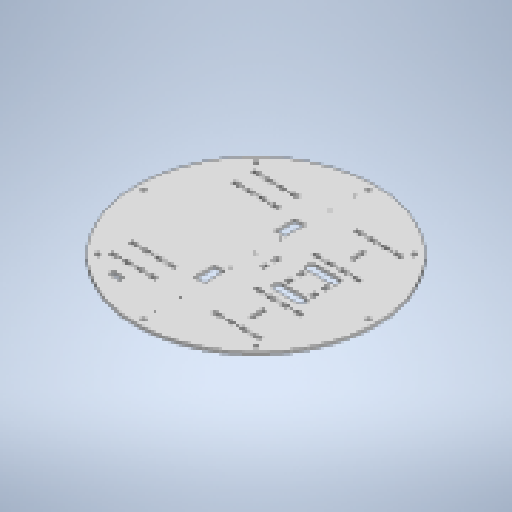
# Autodesk Inventor part: Osn. platform
Saved by Autodesk Inventor 2023.1 (Build 271208000, 208)
## iProperties
Created: 2023-03-13
Part Number: Osn. platform
Material: Типовые
Document SubType Name: Modeling
Designer: User
Density: 1 g/cm^3
Appearance: По умолчанию
Mass: 865.132 g
Surface Area: 3668.91 cm^2
Volume: 865.132 cm^3
Author: User
Autodesk Inventor part; units mm, degrees
(part 1 of 2)
ref_plane "YZ Plane" through (0, 0, 0) normal (1, 0, 0) x (0, 1, 0)
ref_plane "XZ Plane" through (0, 0, 0) normal (0, 1, 0) x (-1, 0, 0)
ref_plane "XY Plane" through (0, 0, 0) normal (0, 0, 1) x (1, 0, 0)
sketch "Основ. платформа" plane through (0, 0, 0) normal (0, 1, 0) x (-1, 0, 0)
  circle A0 centre (0, 0) radius 240
  dimension "d117" = 480
  constraints: 1 centre point, 1 coincident
  measures "d117" diameter of A0
extrude "Осн. платформа" add sketch "Основ. платформа" along normal blind 5
sketch "Эскиз14" plane through (0, 5, 0) normal (0, 1, 0) x (1, 0, 0)
  line L0 (-295.6598, 0) -> (443.256, 0) construction
  line L1 (137.6204, 61.9298) -> (150.9061, 61.9298)
  line L2 (150.9061, 61.9298) -> (150.9061, 55.9298)
  line L3 (137.6204, 55.9298) -> (150.9061, 55.9298)
  line L4 (137.6204, 61.9298) -> (137.6204, 55.9298)
  line L5 (111.049, 61.9298) -> (124.3347, 61.9298)
  line L6 (124.3347, 61.9298) -> (124.3347, 55.9298)
  line L7 (111.049, 55.9298) -> (124.3347, 55.9298)
  line L8 (111.049, 61.9298) -> (111.049, 55.9298)
  line L9 (84.4776, 61.9298) -> (97.7633, 61.9298)
  line L10 (97.7633, 61.9298) -> (97.7633, 55.9298)
  line L11 (84.4776, 55.9298) -> (97.7633, 55.9298)
  line L12 (84.4776, 61.9298) -> (84.4776, 55.9298)
  line L13 (57.9061, 144.9298) -> (71.1919, 144.9298)
  line L14 (71.1919, 144.9298) -> (71.1919, 138.9298)
  line L15 (57.9061, 138.9298) -> (71.1919, 138.9298)
  line L16 (57.9061, 144.9298) -> (57.9061, 138.9298)
  line L17 (84.4776, 144.9298) -> (97.7633, 144.9298)
  line L18 (97.7633, 144.9298) -> (97.7633, 138.9298)
  line L19 (84.4776, 138.9298) -> (97.7633, 138.9298)
  line L20 (84.4776, 144.9298) -> (84.4776, 138.9298)
  line L21 (111.049, 144.9298) -> (124.3347, 144.9298)
  line L22 (124.3347, 144.9298) -> (124.3347, 138.9298)
  line L23 (111.049, 138.9298) -> (124.3347, 138.9298)
  line L24 (111.049, 144.9298) -> (111.049, 138.9298)
  line L25 (137.6204, 144.9298) -> (150.9061, 144.9298)
  line L26 (150.9061, 144.9298) -> (150.9061, 138.9298)
  line L27 (137.6204, 138.9298) -> (150.9061, 138.9298)
  line L28 (137.6204, 144.9298) -> (137.6204, 138.9298)
  line L29 (101.4061, 87.5965) -> (101.4061, 113.2631)
  line L30 (101.4061, 113.2631) -> (107.4061, 113.2631)
  line L31 (107.4061, 113.2631) -> (107.4061, 87.5965)
  line L32 (107.4061, 87.5965) -> (101.4061, 87.5965)
  line L33 (57.9061, 61.9298) -> (71.1919, 61.9298)
  line L34 (71.1919, 61.9298) -> (71.1919, 55.9298)
  line L35 (57.9061, 55.9298) -> (71.1919, 55.9298)
  line L36 (57.9061, 61.9298) -> (57.9061, 55.9298)
  line L37 (-58.1024, 138.9298) -> (-70.9595, 138.9298)
  line L38 (-70.9595, 138.9298) -> (-70.9595, 144.9298)
  line L39 (-58.1024, 144.9298) -> (-70.9595, 144.9298)
  line L40 (-58.1024, 138.9298) -> (-58.1024, 144.9298)
  line L41 (-83.8167, 138.9298) -> (-96.6738, 138.9298)
  line L42 (-96.6738, 138.9298) -> (-96.6738, 144.9298)
  line L43 (-83.8167, 144.9298) -> (-96.6738, 144.9298)
  line L44 (-83.8167, 138.9298) -> (-83.8167, 144.9298)
  line L45 (-109.531, 138.9298) -> (-122.3881, 138.9298)
  line L46 (-122.3881, 138.9298) -> (-122.3881, 144.9298)
  line L47 (-109.531, 144.9298) -> (-122.3881, 144.9298)
  line L48 (-109.531, 138.9298) -> (-109.531, 144.9298)
  line L49 (-135.2452, 140.1831) -> (-148.1024, 140.1831)
  line L50 (-148.1024, 140.1831) -> (-148.1024, 146.1831)
  line L51 (-135.2452, 146.1831) -> (-148.1024, 146.1831)
  line L52 (-135.2452, 140.1831) -> (-135.2452, 146.1831)
  line L53 (-58.1024, 144.9298) -> (-148.1024, 144.9298) construction
  line L54 (-148.1024, 100.7298) -> (-58.1024, 100.7298) construction
  line L55 (137.6204, 138.9298) -> (124.3347, 144.9298) construction
  circle A0 centre (130.9776, 141.9298) radius 1.5
  circle A1 centre (104.2556, 141.9298) radius 1.5
  circle A2 centre (77.5336, 141.9298) radius 1.5
  circle A3 centre (130.9776, 58.9298) radius 1.5
  circle A4 centre (104.2556, 58.9298) radius 1.5
  circle A5 centre (77.5336, 58.9298) radius 1.5
  line L56 (-70.9595, 138.9298) -> (-83.8167, 144.9298) construction
  circle A6 centre (-77.3881, 141.9298) radius 1.5
  circle A7 centre (-103.2571, 141.9298) radius 1.5
  circle A8 centre (-129.1261, 141.9298) radius 1.5
  line L57 (-122.3881, 106.7298) -> (-122.3881, 100.7298)
  line L58 (-109.531, 100.7298) -> (-122.3881, 100.7298)
  line L59 (-109.531, 106.7298) -> (-109.531, 100.7298)
  line L60 (-109.531, 106.7298) -> (-122.3881, 106.7298)
  line L61 (-83.8167, 106.7298) -> (-96.6738, 106.7298)
  line L62 (-70.9595, 106.7298) -> (-70.9595, 100.7298)
  line L63 (-58.1024, 100.7298) -> (-70.9595, 100.7298)
  circle A9 centre (-103.2571, 103.7298) radius 1.5
  circle A10 centre (-129.1261, 103.7298) radius 1.5
  line L64 (-135.2452, 106.7298) -> (-135.2452, 100.7298)
  line L65 (-148.1024, 106.7298) -> (-148.1024, 100.7298)
  line L66 (-135.2452, 100.7298) -> (-148.1024, 100.7298)
  line L67 (-135.2452, 106.7298) -> (-148.1024, 106.7298)
  line L68 (-58.1024, 106.7298) -> (-70.9595, 106.7298)
  line L69 (-58.1024, 106.7298) -> (-58.1024, 100.7298)
  line L70 (-96.6738, 106.7298) -> (-96.6738, 100.7298)
  line L71 (-83.8167, 100.7298) -> (-96.6738, 100.7298)
  line L72 (-83.8167, 106.7298) -> (-83.8167, 100.7298)
  circle A11 centre (-77.3881, 103.7298) radius 1.5
  line L73 (111.049, -61.9298) -> (124.3347, -61.9298)
  line L74 (111.049, -61.9298) -> (111.049, -55.9298)
  line L75 (97.7633, -61.9298) -> (97.7633, -55.9298)
  line L76 (71.1919, -61.9298) -> (71.1919, -55.9298)
  line L77 (57.9061, -61.9298) -> (57.9061, -55.9298)
  line L78 (57.9061, -55.9298) -> (71.1919, -55.9298)
  line L79 (57.9061, -61.9298) -> (71.1919, -61.9298)
  line L80 (107.4061, -87.5965) -> (101.4061, -87.5965)
  line L81 (101.4061, -87.5965) -> (101.4061, -113.2631)
  line L82 (107.4061, -113.2631) -> (107.4061, -87.5965)
  line L83 (57.9061, -138.9298) -> (71.1919, -138.9298)
  line L84 (101.4061, -113.2631) -> (107.4061, -113.2631)
  line L85 (84.4776, -138.9298) -> (97.7633, -138.9298)
  line L86 (84.4776, -144.9298) -> (84.4776, -138.9298)
  line L87 (84.4776, -144.9298) -> (97.7633, -144.9298)
  line L88 (97.7633, -144.9298) -> (97.7633, -138.9298)
  line L89 (111.049, -144.9298) -> (111.049, -138.9298)
  line L90 (111.049, -138.9298) -> (124.3347, -138.9298)
  line L91 (111.049, -144.9298) -> (124.3347, -144.9298)
  line L92 (124.3347, -144.9298) -> (124.3347, -138.9298)
  line L93 (137.6204, -61.9298) -> (150.9061, -61.9298)
  line L94 (150.9061, -61.9298) -> (150.9061, -55.9298)
  line L95 (137.6204, -55.9298) -> (150.9061, -55.9298)
  line L96 (137.6204, -61.9298) -> (137.6204, -55.9298)
  circle A12 centre (130.9776, -58.9298) radius 1.5
  line L97 (137.6204, -144.9298) -> (137.6204, -138.9298)
  line L98 (137.6204, -144.9298) -> (150.9061, -144.9298)
  line L99 (150.9061, -144.9298) -> (150.9061, -138.9298)
  line L100 (137.6204, -138.9298) -> (150.9061, -138.9298)
  line L101 (124.3347, -61.9298) -> (124.3347, -55.9298)
  line L102 (111.049, -55.9298) -> (124.3347, -55.9298)
  line L103 (84.4776, -61.9298) -> (97.7633, -61.9298)
  line L104 (84.4776, -55.9298) -> (97.7633, -55.9298)
  line L105 (84.4776, -61.9298) -> (84.4776, -55.9298)
  line L106 (71.1919, -144.9298) -> (71.1919, -138.9298)
  line L107 (57.9061, -144.9298) -> (71.1919, -144.9298)
  line L108 (57.9061, -144.9298) -> (57.9061, -138.9298)
  line L109 (-58.1024, -100.7298) -> (-70.9595, -100.7298)
  line L110 (-70.9595, -106.7298) -> (-70.9595, -100.7298)
  line L111 (-135.2452, -140.1831) -> (-135.2452, -146.1831)
  line L112 (-135.2452, -140.1831) -> (-148.1024, -140.1831)
  line L113 (-148.1024, -140.1831) -> (-148.1024, -146.1831)
  line L114 (-135.2452, -146.1831) -> (-148.1024, -146.1831)
  line L115 (-96.6738, -138.9298) -> (-96.6738, -144.9298)
  line L116 (-83.8167, -138.9298) -> (-96.6738, -138.9298)
  line L117 (-109.531, -138.9298) -> (-109.531, -144.9298)
  line L118 (-83.8167, -144.9298) -> (-96.6738, -144.9298)
  line L119 (-83.8167, -138.9298) -> (-83.8167, -144.9298)
  circle A13 centre (-129.1261, -141.9298) radius 1.5
  circle A14 centre (-129.1261, -103.7298) radius 1.5
  line L120 (-122.3881, -138.9298) -> (-122.3881, -144.9298)
  line L121 (-122.3881, -106.7298) -> (-122.3881, -100.7298)
  line L122 (-109.531, -144.9298) -> (-122.3881, -144.9298)
  line L123 (-109.531, -100.7298) -> (-122.3881, -100.7298)
  line L124 (-109.531, -138.9298) -> (-122.3881, -138.9298)
  line L125 (-109.531, -106.7298) -> (-122.3881, -106.7298)
  line L126 (-148.1024, -100.7298) -> (-58.1024, -100.7298) construction
  line L127 (-58.1024, -144.9298) -> (-148.1024, -144.9298) construction
  line L128 (-70.9595, -138.9298) -> (-70.9595, -144.9298)
  line L129 (-58.1024, -144.9298) -> (-70.9595, -144.9298)
  line L130 (-109.531, -106.7298) -> (-109.531, -100.7298)
  circle A15 centre (-103.2571, -141.9298) radius 1.5
  line L131 (-135.2452, -106.7298) -> (-135.2452, -100.7298)
  line L132 (-135.2452, -106.7298) -> (-148.1024, -106.7298)
  line L133 (-148.1024, -106.7298) -> (-148.1024, -100.7298)
  line L134 (-135.2452, -100.7298) -> (-148.1024, -100.7298)
  circle A16 centre (77.5336, -58.9298) radius 1.5
  line L135 (-58.1024, -106.7298) -> (-70.9595, -106.7298)
  line L136 (-58.1024, -106.7298) -> (-58.1024, -100.7298)
  line L137 (-58.1024, -138.9298) -> (-70.9595, -138.9298)
  line L138 (-58.1024, -138.9298) -> (-58.1024, -144.9298)
  circle A17 centre (130.9776, -141.9298) radius 1.5
  line L139 (137.6204, -138.9298) -> (124.3347, -144.9298) construction
  circle A18 centre (104.2556, -141.9298) radius 1.5
  circle A19 centre (77.5336, -141.9298) radius 1.5
  circle A20 centre (104.2556, -58.9298) radius 1.5
  line L140 (-70.9595, -138.9298) -> (-83.8167, -144.9298) construction
  circle A21 centre (-77.3881, -141.9298) radius 1.5
  circle A22 centre (-103.2571, -103.7298) radius 1.5
  line L141 (-96.6738, -106.7298) -> (-96.6738, -100.7298)
  line L142 (-83.8167, -100.7298) -> (-96.6738, -100.7298)
  line L143 (-83.8167, -106.7298) -> (-83.8167, -100.7298)
  line L144 (-83.8167, -106.7298) -> (-96.6738, -106.7298)
  circle A23 centre (-77.3881, -103.7298) radius 1.5
  point P0 (0, 0)
  point P1 (-58.1024, 122.8298)
  point P2 (-148.1024, 122.8298)
  point P3 (-148.1024, 100.7298)
  point P4 (-148.1024, -122.8298)
  point P5 (-58.1024, -122.8298)
  point P6 (-148.1024, -100.7298)
  constraints: 290 end point, 85 symmetric about line, 24 centre point, 1 horizontal, 12 other
extrude "Выдавливание9" cut sketch "Эскиз14" against normal up to surface (5 mm away)
sketch "Эскиз16" plane through (0, 5, 0) normal (0, 1, 0) x (1, 0, 0)
  line L0 (-17, -32) -> (-7, -32) construction
  line L1 (-7, -32) -> (-7, -25) construction
  line L2 (-7, -25) -> (-17, -25) construction
  line L3 (-17, -25) -> (-17, -32) construction
  line L4 (66.5859, 0) -> (-61.9521, 0) construction
  line L5 (0, -82.102) -> (0, 52.9941) construction
  line L6 (-17, -75) -> (-17, -82) construction
  line L7 (-17, -82) -> (-7, -82) construction
  line L8 (-7, -82) -> (-7, -75) construction
  line L9 (-7, -75) -> (-17, -75) construction
  line L10 (-17, -125) -> (-17, -132) construction
  line L11 (-17, -132) -> (-7, -132) construction
  line L12 (-7, -132) -> (-7, -125) construction
  line L13 (-7, -125) -> (-17, -125) construction
  line L14 (7, -25) -> (7, -32) construction
  line L15 (7, -32) -> (17, -32) construction
  line L16 (17, -32) -> (17, -25) construction
  line L17 (17, -25) -> (7, -25) construction
  line L18 (7, -75) -> (7, -82) construction
  line L19 (7, -82) -> (17, -82) construction
  line L20 (17, -82) -> (17, -75) construction
  line L21 (17, -75) -> (7, -75) construction
  line L22 (7, -125) -> (7, -132) construction
  line L23 (7, -132) -> (17, -132) construction
  line L24 (17, -132) -> (17, -125) construction
  line L25 (17, -125) -> (7, -125) construction
  line L26 (32, -7) -> (25, -7)
  line L27 (25, -7) -> (25, -17)
  line L28 (25, -17) -> (32, -17)
  line L29 (32, -17) -> (32, -7)
  line L30 (32, -7) -> (25, -17) construction
  line L31 (25, -7) -> (32, -17) construction
  line L32 (75, -17) -> (82, -17)
  line L33 (82, -17) -> (82, -7)
  line L34 (82, -7) -> (75, -7)
  line L35 (75, -7) -> (75, -17)
  line L36 (125, -17) -> (132, -17)
  line L37 (132, -17) -> (132, -7)
  line L38 (132, -7) -> (125, -7)
  line L39 (125, -7) -> (125, -17)
  line L40 (25, 7) -> (32, 7)
  line L41 (32, 7) -> (32, 17)
  line L42 (32, 17) -> (25, 17)
  line L43 (25, 17) -> (25, 7)
  line L44 (75, 7) -> (82, 7)
  line L45 (82, 7) -> (82, 17)
  line L46 (82, 17) -> (75, 17)
  line L47 (75, 17) -> (75, 7)
  line L48 (125, 7) -> (132, 7)
  line L49 (132, 7) -> (132, 17)
  line L50 (132, 17) -> (125, 17)
  line L51 (125, 17) -> (125, 7)
  circle A0 centre (104.2556, -58.9298) radius 1.5 construction
  circle A1 centre (130.9776, -58.9298) radius 1.5 construction
  line L52 (125.6303, -33.4298) -> (77.5364, -33.4298) construction
  line L53 (125.6303, -24.4298) -> (77.5364, -24.4298)
  line L54 (77.5364, -42.4298) -> (125.6303, -42.4298)
  arc A2 (125.6303, -42.4298) -> (125.6303, -24.4298) centre (125.6303, -33.4298) ccw
  arc A3 (77.5364, -24.4298) -> (77.5364, -42.4298) centre (77.5364, -33.4298) ccw
  line L55 (125.6303, 33.4298) -> (77.5364, 33.4298) construction
  line L56 (125.6303, 24.4298) -> (77.5364, 24.4298)
  line L57 (77.5364, 42.4298) -> (125.6303, 42.4298)
  arc A4 (125.6303, 24.4298) -> (125.6303, 42.4298) centre (125.6303, 33.4298) ccw
  arc A5 (77.5364, 42.4298) -> (77.5364, 24.4298) centre (77.5364, 33.4298) ccw
  circle A6 centre (-225.3213, 0) radius 4
  circle A7 centre (-159.3262, -159.3262) radius 4
  circle A8 centre (0, -225.3213) radius 4
  circle A9 centre (159.3262, -159.3262) radius 4
  circle A10 centre (225.3213, 0) radius 4
  circle A11 centre (159.3262, 159.3262) radius 4
  circle A12 centre (0, 225.3213) radius 4
  circle A13 centre (-159.3262, 159.3262) radius 4
  line L58 (-22, 32) -> (22, 32) construction
  line L59 (32, 22) -> (32, -22) construction
  line L60 (22, -32) -> (-22, -32) construction
  line L61 (-32, -22) -> (-32, 22) construction
  line L62 (-32, 32) -> (32, -32) construction
  line L63 (32, 32) -> (-32, -32) construction
  arc A14 (-22, 32) -> (-32, 22) centre (-22, 22) ccw construction
  arc A15 (-32, -22) -> (-22, -32) centre (-22, -22) ccw construction
  arc A16 (22, -32) -> (32, -22) centre (22, -22) ccw construction
  arc A17 (32, 22) -> (22, 32) centre (22, 22) ccw construction
  line L64 (-4.1722, 101.2362) -> (-8.7222, 101.2388) construction
  arc A18 (-22.6837, 81.7061) -> (-22.6574, 81.5943) centre (-22.4337, 81.7059) ccw construction
  line L65 (-22.6574, 81.5943) -> (-22.484, 81.247) construction
  line L66 (-22.484, 81.247) -> (-22.6578, 80.8998) construction
  arc A19 (-22.6578, 80.8998) -> (-22.6843, 80.7881) centre (-22.4343, 80.7879) ccw construction
  line L67 (-22.6843, 80.7881) -> (-22.6876, 75.1971) construction
  arc A20 (-22.6876, 75.1971) -> (-22.4377, 74.9469) centre (-22.4376, 75.1969) ccw construction
  line L68 (-22.4377, 74.9469) -> (-22.0877, 74.9467) construction
  line L69 (-22.0877, 74.9467) -> (-22.0879, 74.5667) construction
  arc A21 (-22.0879, 74.5667) -> (-21.8381, 74.3166) centre (-21.8379, 74.5666) ccw construction
  line L70 (-21.8381, 74.3166) -> (-20.9381, 74.316) construction
  arc A22 (-20.9381, 74.316) -> (-20.6879, 74.5659) centre (-20.9379, 74.566) ccw construction
  line L71 (-20.6879, 74.5659) -> (-20.687, 76.1959) construction
  arc A23 (-20.4368, 76.4457) -> (-20.687, 76.1959) centre (-20.437, 76.1957) ccw construction
  line L72 (-20.4368, 76.4457) -> (-19.291, 76.4451) construction
  arc A24 (-18.5841, 76.1518) -> (-19.291, 76.4451) centre (-19.2916, 75.4451) ccw construction
  line L73 (-18.5841, 76.1518) -> (-17.2736, 74.8397) construction
  arc A25 (-16.6886, 73.4252) -> (-17.2736, 74.8397) centre (-18.6886, 73.4263) ccw construction
  line L74 (-16.6886, 73.4252) -> (-16.6896, 71.7026) construction
  arc A26 (-16.6896, 71.7026) -> (-16.6633, 71.5907) centre (-16.4396, 71.7024) ccw construction
  line L75 (-16.6633, 71.5907) -> (-16.4899, 71.2434) construction
  line L76 (-16.4899, 71.2434) -> (-16.6637, 70.8963) construction
  arc A27 (-16.6637, 70.8963) -> (-16.6902, 70.7845) centre (-16.4402, 70.7843) ccw construction
  line L77 (-16.6902, 70.7845) -> (-16.6912, 69.0619) construction
  arc A28 (-17.2778, 67.648) -> (-16.6912, 69.0619) centre (-18.6912, 69.0631) ccw construction
  line L78 (-17.2778, 67.648) -> (-18.5898, 66.3375) construction
  arc A29 (-19.2971, 66.0451) -> (-18.5898, 66.3375) centre (-19.2965, 67.0451) ccw construction
  line L79 (-19.2971, 66.0451) -> (-20.443, 66.0457) construction
  arc A30 (-20.6928, 66.2959) -> (-20.443, 66.0457) centre (-20.4428, 66.2957) ccw construction
  line L80 (-20.6928, 66.2959) -> (-20.6919, 67.9259) construction
  arc A31 (-20.6919, 67.9259) -> (-20.9417, 68.176) centre (-20.9419, 67.926) ccw construction
  line L81 (-20.9417, 68.176) -> (-21.8417, 68.1766) construction
  arc A32 (-21.8417, 68.1766) -> (-22.0919, 67.9267) centre (-21.8419, 67.9266) ccw construction
  line L82 (-22.0919, 67.9267) -> (-22.0921, 67.5467) construction
  line L83 (-22.0921, 67.5467) -> (-22.4421, 67.5469) construction
  arc A33 (-22.4421, 67.5469) -> (-22.6922, 67.2971) centre (-22.4422, 67.2969) ccw construction
  line L84 (-22.6922, 67.2971) -> (-22.6949, 62.7471) construction
  arc A34 (-22.6949, 62.7471) -> (-21.1958, 61.2462) centre (-21.1949, 62.7462) ccw construction
  line L85 (-21.1958, 61.2462) -> (-16.6458, 61.2435) construction
  arc A35 (-16.6458, 61.2435) -> (-16.3956, 61.4934) centre (-16.6456, 61.4935) ccw construction
  line L86 (-16.3956, 61.4934) -> (-16.3954, 61.8434) construction
  line L87 (-16.3954, 61.8434) -> (-16.0154, 61.8431) construction
  arc A36 (-16.0154, 61.8431) -> (-15.7653, 62.093) centre (-16.0153, 62.0931) ccw construction
  line L88 (-15.7653, 62.093) -> (-15.7648, 62.993) construction
  arc A37 (-15.7648, 62.993) -> (-15.9008, 63.2431) centre (-16.0623, 62.9932) ccw construction
  line L89 (-15.9008, 63.2431) -> (-17.6446, 63.2441) construction
  arc A38 (-17.8945, 63.4942) -> (-17.6446, 63.2441) centre (-17.6445, 63.4941) ccw construction
  line L90 (-17.8945, 63.4942) -> (-17.8938, 64.6401) construction
  arc A39 (-17.6005, 65.347) -> (-17.8938, 64.6401) centre (-16.8938, 64.6395) ccw construction
  line L91 (-17.6005, 65.347) -> (-16.2884, 66.6575) construction
  arc A40 (-14.8739, 67.2425) -> (-16.2884, 66.6575) centre (-14.875, 65.2425) ccw construction
  line L92 (-14.8739, 67.2425) -> (-13.1513, 67.2414) construction
  arc A41 (-13.1513, 67.2414) -> (-13.0394, 67.2678) centre (-13.1511, 67.4914) ccw construction
  line L93 (-13.0394, 67.2678) -> (-12.6921, 67.4412) construction
  line L94 (-12.6921, 67.4412) -> (-12.345, 67.2674) construction
  arc A42 (-12.345, 67.2674) -> (-12.2332, 67.2409) centre (-12.2331, 67.4909) ccw construction
  line L95 (-12.2332, 67.2409) -> (-10.5106, 67.2399) construction
  arc A43 (-9.0968, 66.6533) -> (-10.5106, 67.2399) centre (-10.5118, 65.2399) ccw construction
  line L96 (-9.0968, 66.6533) -> (-7.7863, 65.3412) construction
  arc A44 (-7.4938, 64.6339) -> (-7.7863, 65.3412) centre (-8.4938, 64.6345) ccw construction
  line L97 (-7.4938, 64.6339) -> (-7.4945, 63.4881) construction
  arc A45 (-7.7446, 63.2383) -> (-7.4945, 63.4881) centre (-7.7445, 63.4883) ccw construction
  line L98 (-7.7446, 63.2383) -> (-9.5773, 63.2393) construction
  arc A46 (-9.5773, 63.2393) -> (-9.6248, 62.9894) centre (-8.9399, 62.989) ccw construction
  line L99 (-9.6248, 62.9894) -> (-9.6253, 62.0894) construction
  arc A47 (-9.6253, 62.0894) -> (-9.3754, 61.8392) centre (-9.3753, 62.0892) ccw construction
  line L100 (-9.3754, 61.8392) -> (-8.9954, 61.839) construction
  line L101 (-8.9954, 61.839) -> (-8.9956, 61.489) construction
  arc A48 (-8.9956, 61.489) -> (-8.7458, 61.2389) centre (-8.7456, 61.4889) ccw construction
  line L102 (-8.7458, 61.2389) -> (-4.1958, 61.2362) construction
  arc A49 (-4.1958, 61.2362) -> (-2.6949, 62.7353) centre (-4.1949, 62.7362) ccw construction
  line L103 (-2.6949, 62.7353) -> (-2.6922, 67.2853) construction
  arc A50 (-2.6922, 67.2853) -> (-2.9421, 67.5354) centre (-2.9422, 67.2854) ccw construction
  line L104 (-2.9421, 67.5354) -> (-3.2921, 67.5356) construction
  line L105 (-3.2921, 67.5356) -> (-3.2919, 67.9156) construction
  arc A51 (-3.2919, 67.9156) -> (-3.5417, 68.1658) centre (-3.5419, 67.9158) ccw construction
  line L106 (-3.5417, 68.1658) -> (-4.4417, 68.1663) construction
  arc A52 (-4.4417, 68.1663) -> (-4.6919, 67.9165) centre (-4.4419, 67.9163) ccw construction
  line L107 (-4.6919, 67.9165) -> (-4.6928, 66.2865) construction
  arc A53 (-4.943, 66.0366) -> (-4.6928, 66.2865) centre (-4.9428, 66.2866) ccw construction
  line L108 (-4.943, 66.0366) -> (-6.0888, 66.0373) construction
  arc A54 (-6.7957, 66.3306) -> (-6.0888, 66.0373) centre (-6.0882, 67.0373) ccw construction
  line L109 (-6.7957, 66.3306) -> (-8.1062, 67.6426) construction
  arc A55 (-8.6912, 69.0572) -> (-8.1062, 67.6426) centre (-6.6912, 69.056) ccw construction
  line L110 (-8.6912, 69.0572) -> (-8.6902, 70.7798) construction
  arc A56 (-8.6902, 70.7798) -> (-8.7165, 70.8916) centre (-8.9402, 70.78) ccw construction
  line L111 (-8.7165, 70.8916) -> (-8.8899, 71.2389) construction
  line L112 (-8.8899, 71.2389) -> (-8.7161, 71.586) construction
  arc A57 (-8.7161, 71.586) -> (-8.6896, 71.6978) centre (-8.9396, 71.698) ccw construction
  line L113 (-8.6896, 71.6978) -> (-8.6886, 73.4204) construction
  arc A58 (-8.102, 74.8343) -> (-8.6886, 73.4204) centre (-6.6886, 73.4193) ccw construction
  line L114 (-8.102, 74.8343) -> (-6.7899, 76.1448) construction
  arc A59 (-6.0827, 76.4373) -> (-6.7899, 76.1448) centre (-6.0833, 75.4373) ccw construction
  line L115 (-6.0827, 76.4373) -> (-4.9368, 76.4366) construction
  arc A60 (-4.687, 76.1865) -> (-4.9368, 76.4366) centre (-4.937, 76.1866) ccw construction
  line L116 (-4.687, 76.1865) -> (-4.6879, 74.5565) construction
  arc A61 (-4.6879, 74.5565) -> (-4.4381, 74.3063) centre (-4.4379, 74.5563) ccw construction
  line L117 (-4.4381, 74.3063) -> (-3.5381, 74.3058) construction
  arc A62 (-3.5381, 74.3058) -> (-3.2879, 74.5556) centre (-3.5379, 74.5558) ccw construction
  line L118 (-3.2879, 74.5556) -> (-3.2877, 74.9356) construction
  line L119 (-3.2877, 74.9356) -> (-2.9377, 74.9354) construction
  arc A63 (-2.9377, 74.9354) -> (-2.6876, 75.1853) centre (-2.9376, 75.1854) ccw construction
  line L120 (-2.6876, 75.1853) -> (-2.6843, 80.7763) construction
  arc A64 (-2.6843, 80.7763) -> (-2.7106, 80.8881) centre (-2.9343, 80.7764) ccw construction
  line L121 (-2.7106, 80.8881) -> (-2.884, 81.2354) construction
  line L122 (-2.884, 81.2354) -> (-2.7102, 81.5825) construction
  arc A65 (-2.7102, 81.5825) -> (-2.6837, 81.6943) centre (-2.9337, 81.6944) ccw construction
  line L123 (-2.6837, 81.6943) -> (-2.6804, 87.2853) construction
  arc A66 (-2.6804, 87.2853) -> (-2.9303, 87.5354) centre (-2.9304, 87.2854) ccw construction
  line L124 (-2.9303, 87.5354) -> (-3.2803, 87.5356) construction
  line L125 (-3.2803, 87.5356) -> (-3.2801, 87.9156) construction
  arc A67 (-3.2801, 87.9156) -> (-3.5299, 88.1658) centre (-3.5301, 87.9158) ccw construction
  line L126 (-3.5299, 88.1658) -> (-4.4299, 88.1663) construction
  arc A68 (-4.4299, 88.1663) -> (-4.6801, 87.9165) centre (-4.4301, 87.9163) ccw construction
  line L127 (-4.6801, 87.9165) -> (-4.681, 86.2865) construction
  arc A69 (-4.9312, 86.0366) -> (-4.681, 86.2865) centre (-4.931, 86.2866) ccw construction
  line L128 (-4.9312, 86.0366) -> (-6.077, 86.0373) construction
  arc A70 (-6.7839, 86.3306) -> (-6.077, 86.0373) centre (-6.0764, 87.0373) ccw construction
  line L129 (-6.7839, 86.3306) -> (-8.0944, 87.6426) construction
  arc A71 (-8.6794, 89.0572) -> (-8.0944, 87.6426) centre (-6.6794, 89.056) ccw construction
  line L130 (-8.6794, 89.0572) -> (-8.6784, 90.7798) construction
  arc A72 (-8.6784, 90.7798) -> (-8.7047, 90.8916) centre (-8.9284, 90.7799) ccw construction
  line L131 (-8.7047, 90.8916) -> (-8.8781, 91.2389) construction
  line L132 (-8.8781, 91.2389) -> (-8.7043, 91.586) construction
  arc A73 (-8.7043, 91.586) -> (-8.6778, 91.6978) centre (-8.9278, 91.698) ccw construction
  line L133 (-8.6778, 91.6978) -> (-8.6768, 93.4204) construction
  arc A74 (-8.0902, 94.8343) -> (-8.6768, 93.4204) centre (-6.6768, 93.4193) ccw construction
  line L134 (-8.0902, 94.8343) -> (-6.7782, 96.1448) construction
  arc A75 (-6.0709, 96.4373) -> (-6.7782, 96.1448) centre (-6.0715, 95.4373) ccw construction
  line L135 (-6.0709, 96.4373) -> (-4.925, 96.4366) construction
  arc A76 (-4.6752, 96.1865) -> (-4.925, 96.4366) centre (-4.9252, 96.1866) ccw construction
  line L136 (-4.6752, 96.1865) -> (-4.6761, 94.5565) construction
  arc A77 (-4.6761, 94.5565) -> (-4.4263, 94.3063) centre (-4.4261, 94.5563) ccw construction
  line L137 (-4.4263, 94.3063) -> (-3.5263, 94.3058) construction
  arc A78 (-3.5263, 94.3058) -> (-3.2761, 94.5556) centre (-3.5261, 94.5558) ccw construction
  line L138 (-3.2761, 94.5556) -> (-3.2759, 94.9356) construction
  line L139 (-3.2759, 94.9356) -> (-2.9259, 94.9354) construction
  arc A79 (-2.9259, 94.9354) -> (-2.6758, 95.1853) centre (-2.9258, 95.1854) ccw construction
  line L140 (-2.6758, 95.1853) -> (-2.6731, 99.7353) construction
  arc A80 (-2.6731, 99.7353) -> (-4.1722, 101.2362) centre (-4.1731, 99.7362) ccw construction
  line L141 (-4.1722, 101.2362) -> (-8.7222, 101.2388) construction
  arc A81 (-8.7222, 101.2388) -> (-8.9723, 100.989) centre (-8.7223, 100.9888) ccw construction
  line L142 (-8.9723, 100.989) -> (-8.9726, 100.639) construction
  line L143 (-8.9726, 100.639) -> (-9.3526, 100.6392) construction
  arc A82 (-9.3526, 100.6392) -> (-9.6027, 100.3894) centre (-9.3527, 100.3892) ccw construction
  line L144 (-9.6027, 100.3894) -> (-9.6032, 99.4894) construction
  arc A83 (-9.6032, 99.4894) -> (-9.3534, 99.2392) centre (-9.3532, 99.4892) ccw construction
  line L145 (-9.3534, 99.2392) -> (-7.7234, 99.2383) construction
  arc A84 (-7.4735, 98.9881) -> (-7.7234, 99.2383) centre (-7.7235, 98.9883) ccw construction
  line L146 (-7.4735, 98.9881) -> (-7.4742, 97.8423) construction
  arc A85 (-7.7675, 97.1353) -> (-7.4742, 97.8423) centre (-8.4742, 97.8429) ccw construction
  line L147 (-7.7675, 97.1353) -> (-9.0796, 95.8248) construction
  arc A86 (-10.4941, 95.2399) -> (-9.0796, 95.8248) centre (-10.4929, 97.2399) ccw construction
  line L148 (-10.4941, 95.2399) -> (-12.2167, 95.2409) construction
  arc A87 (-12.2167, 95.2409) -> (-12.3285, 95.2146) centre (-12.2169, 94.9909) ccw construction
  line L149 (-12.3285, 95.2146) -> (-12.6759, 95.0412) construction
  line L150 (-12.6759, 95.0412) -> (-13.023, 95.215) construction
  arc A88 (-13.023, 95.215) -> (-13.1348, 95.2414) centre (-13.1349, 94.9914) ccw construction
  line L151 (-13.1348, 95.2414) -> (-14.8574, 95.2425) construction
  arc A89 (-16.2712, 95.8291) -> (-14.8574, 95.2425) centre (-14.8562, 97.2425) ccw construction
  line L152 (-16.2712, 95.8291) -> (-17.5817, 97.1411) construction
  arc A90 (-17.8742, 97.8484) -> (-17.5817, 97.1411) centre (-16.8742, 97.8478) ccw construction
  line L153 (-17.8742, 97.8484) -> (-17.8735, 98.9942) construction
  arc A91 (-17.6234, 99.2441) -> (-17.8735, 98.9942) centre (-17.6235, 98.9941) ccw construction
  line L154 (-17.6234, 99.2441) -> (-15.9934, 99.2431) construction
  arc A92 (-15.9934, 99.2431) -> (-15.7432, 99.493) centre (-15.9932, 99.4931) ccw construction
  line L155 (-15.7432, 99.493) -> (-15.7427, 100.393) construction
  arc A93 (-15.7427, 100.393) -> (-15.9926, 100.6431) centre (-15.9927, 100.3931) ccw construction
  line L156 (-15.9926, 100.6431) -> (-16.3726, 100.6434) construction
  line L157 (-16.3726, 100.6434) -> (-16.3723, 100.9934) construction
  arc A94 (-16.3723, 100.9934) -> (-16.4557, 101.2434) centre (-16.7884, 100.9936) ccw construction
  line L158 (-16.4557, 101.2434) -> (-21.5905, 101.2464) construction
  arc A95 (-21.5905, 101.2464) -> (-22.6731, 99.7471) centre (-21.0922, 99.7461) ccw construction
  line L159 (-22.6731, 99.7471) -> (-22.6758, 95.1971) construction
  arc A96 (-22.6758, 95.1971) -> (-22.4259, 94.9469) centre (-22.4258, 95.1969) ccw construction
  line L160 (-22.4259, 94.9469) -> (-22.0759, 94.9467) construction
  line L161 (-22.0759, 94.9467) -> (-22.0761, 94.5667) construction
  arc A97 (-22.0761, 94.5667) -> (-21.8263, 94.3166) centre (-21.8261, 94.5666) ccw construction
  line L162 (-21.8263, 94.3166) -> (-20.9263, 94.316) construction
  arc A98 (-20.9263, 94.316) -> (-20.6761, 94.5659) centre (-20.9261, 94.566) ccw construction
  line L163 (-20.6761, 94.5659) -> (-20.6752, 96.1959) construction
  arc A99 (-20.425, 96.4457) -> (-20.6752, 96.1959) centre (-20.4252, 96.1957) ccw construction
  line L164 (-20.425, 96.4457) -> (-19.2792, 96.4451) construction
  arc A100 (-18.5723, 96.1518) -> (-19.2792, 96.4451) centre (-19.2798, 95.4451) ccw construction
  line L165 (-18.5723, 96.1518) -> (-17.2618, 94.8397) construction
  arc A101 (-16.6768, 93.4252) -> (-17.2618, 94.8397) centre (-18.6768, 93.4263) ccw construction
  line L166 (-16.6768, 93.4252) -> (-16.6778, 91.7026) construction
  arc A102 (-16.6778, 91.7026) -> (-16.6515, 91.5907) centre (-16.4278, 91.7024) ccw construction
  line L167 (-16.6515, 91.5907) -> (-16.4781, 91.2434) construction
  line L168 (-16.4781, 91.2434) -> (-16.6519, 90.8963) construction
  arc A103 (-16.6519, 90.8963) -> (-16.6784, 90.7845) centre (-16.4284, 90.7844) ccw construction
  line L169 (-16.6784, 90.7845) -> (-16.6794, 89.0619) construction
  arc A104 (-17.266, 87.648) -> (-16.6794, 89.0619) centre (-18.6794, 89.0631) ccw construction
  line L170 (-17.266, 87.648) -> (-18.5781, 86.3375) construction
  arc A105 (-19.2853, 86.0451) -> (-18.5781, 86.3375) centre (-19.2847, 87.0451) ccw construction
  line L171 (-19.2853, 86.0451) -> (-20.4312, 86.0457) construction
  arc A106 (-20.681, 86.2959) -> (-20.4312, 86.0457) centre (-20.431, 86.2957) ccw construction
  line L172 (-20.681, 86.2959) -> (-20.6801, 87.9259) construction
  arc A107 (-20.6801, 87.9259) -> (-20.9299, 88.176) centre (-20.9301, 87.926) ccw construction
  line L173 (-20.9299, 88.176) -> (-21.8299, 88.1766) construction
  arc A108 (-21.8299, 88.1766) -> (-22.0801, 87.9267) centre (-21.8301, 87.9266) ccw construction
  line L174 (-22.0801, 87.9267) -> (-22.0803, 87.5467) construction
  line L175 (-22.0803, 87.5467) -> (-22.4303, 87.5469) construction
  arc A109 (-22.4303, 87.5469) -> (-22.6804, 87.2971) centre (-22.4304, 87.2969) ccw construction
  line L176 (-22.6804, 87.2971) -> (-22.6837, 81.7061) construction
  line L177 (-20.586, 77.8958) -> (-18.6895, 77.8947) construction
  arc A110 (-21.1856, 78.4962) -> (-20.586, 77.8958) centre (-20.5856, 78.4958) ccw construction
  line L178 (-21.1846, 80.1692) -> (-21.1856, 78.4962) construction
  arc A111 (-21.1846, 80.1692) -> (-21.1834, 82.3232) centre (-23.984, 81.2478) ccw construction
  line L179 (-21.1824, 83.9962) -> (-21.1834, 82.3232) construction
  arc A112 (-20.582, 84.5958) -> (-21.1824, 83.9962) centre (-20.5824, 83.9958) ccw construction
  line L180 (-18.6856, 84.5947) -> (-20.582, 84.5958) construction
  arc A113 (-18.6856, 84.5947) -> (-17.9783, 84.8872) centre (-18.685, 85.5947) ccw construction
  line L181 (-15.9129, 86.9502) -> (-17.9783, 84.8872) construction
  arc A114 (-15.2056, 87.2427) -> (-15.9129, 86.9502) centre (-15.2062, 86.2427) ccw construction
  line L182 (-10.1553, 87.2397) -> (-15.2056, 87.2427) construction
  arc A115 (-9.4484, 86.9464) -> (-10.1553, 87.2397) centre (-10.1559, 86.2397) ccw construction
  line L183 (-7.3854, 84.8809) -> (-9.4484, 86.9464) construction
  arc A116 (-7.3854, 84.8809) -> (-6.6785, 84.5876) centre (-6.6779, 85.5877) ccw construction
  line L184 (-4.782, 84.5865) -> (-6.6785, 84.5876) construction
  arc A117 (-4.1824, 83.9862) -> (-4.782, 84.5865) centre (-4.7824, 83.9865) ccw construction
  line L185 (-4.1834, 82.3132) -> (-4.1824, 83.9862) construction
  arc A118 (-4.1834, 82.3132) -> (-4.1846, 80.1591) centre (-1.384, 81.2345) ccw construction
  line L186 (-4.1856, 78.4862) -> (-4.1846, 80.1591) construction
  arc A119 (-4.786, 77.8865) -> (-4.1856, 78.4862) centre (-4.7856, 78.4865) ccw construction
  line L187 (-6.6824, 77.8876) -> (-4.786, 77.8865) construction
  arc A120 (-6.6824, 77.8876) -> (-7.3897, 77.5952) centre (-6.683, 76.8876) ccw construction
  line L188 (-9.4551, 75.5322) -> (-7.3897, 77.5952) construction
  arc A121 (-10.1624, 75.2397) -> (-9.4551, 75.5322) centre (-10.1618, 76.2397) ccw construction
  line L189 (-15.2127, 75.2427) -> (-10.1624, 75.2397) construction
  arc A122 (-15.9196, 75.536) -> (-15.2127, 75.2427) centre (-15.2121, 76.2427) ccw construction
  line L190 (-17.9826, 77.6014) -> (-15.9196, 75.536) construction
  arc A123 (-17.9826, 77.6014) -> (-18.6895, 77.8947) centre (-18.6901, 76.8947) ccw construction
  arc A124 (-10.3229, 70.4366) -> (-10.3219, 69.7902) centre (-9.3761, 70.1148) ccw construction
  arc A125 (-11.2417, 68.8715) -> (-10.3219, 69.7902) centre (-10.7818, 69.3309) ccw construction
  arc A126 (-11.2417, 68.8715) -> (-11.8881, 68.8732) centre (-11.5674, 67.926) ccw construction
  arc A127 (-13.4944, 68.8742) -> (-11.8881, 68.8732) centre (-12.6899, 71.2412) ccw construction
  arc A128 (-13.4944, 68.8742) -> (-14.1409, 68.8732) centre (-13.8163, 67.9274) ccw construction
  arc A129 (-15.0596, 69.793) -> (-14.1409, 68.8732) centre (-14.6002, 69.3331) ccw construction
  arc A130 (-15.0596, 69.793) -> (-15.0578, 70.4394) centre (-16.005, 70.1187) ccw construction
  arc A131 (-15.0569, 72.0457) -> (-15.0578, 70.4394) centre (-12.6899, 71.2412) ccw construction
  arc A132 (-15.0569, 72.0457) -> (-15.0578, 72.6921) centre (-16.0037, 72.3675) ccw construction
  arc A133 (-14.1381, 73.6108) -> (-15.0578, 72.6921) centre (-14.598, 73.1515) ccw construction
  arc A134 (-14.1381, 73.6108) -> (-13.4916, 73.6091) centre (-13.8123, 74.5563) ccw construction
  arc A135 (-11.8853, 73.6082) -> (-13.4916, 73.6091) centre (-12.6899, 71.2412) ccw construction
  arc A136 (-11.8853, 73.6082) -> (-11.2389, 73.6091) centre (-11.5635, 74.555) ccw construction
  arc A137 (-10.3202, 72.6893) -> (-11.2389, 73.6091) centre (-10.7796, 73.1492) ccw construction
  arc A138 (-10.3202, 72.6893) -> (-10.3219, 72.0429) centre (-9.3748, 72.3636) ccw construction
  arc A139 (-10.3229, 70.4366) -> (-10.3219, 72.0429) centre (-12.6899, 71.2412) ccw construction
  arc A140 (-14.1263, 93.6108) -> (-13.4799, 93.6091) centre (-13.8006, 94.5563) ccw construction
  arc A141 (-11.8736, 93.6082) -> (-13.4799, 93.6091) centre (-12.6781, 91.2412) ccw construction
  arc A142 (-11.8736, 93.6082) -> (-11.2271, 93.6091) centre (-11.5517, 94.555) ccw construction
  arc A143 (-10.3084, 92.6893) -> (-11.2271, 93.6091) centre (-10.7678, 93.1492) ccw construction
  arc A144 (-10.3084, 92.6893) -> (-10.3101, 92.0429) centre (-9.363, 92.3636) ccw construction
  arc A145 (-10.3111, 90.4366) -> (-10.3101, 92.0429) centre (-12.6781, 91.2412) ccw construction
  arc A146 (-10.3111, 90.4366) -> (-10.3101, 89.7902) centre (-9.3643, 90.1148) ccw construction
  arc A147 (-11.2299, 88.8715) -> (-10.3101, 89.7902) centre (-10.77, 89.3309) ccw construction
  arc A148 (-11.2299, 88.8715) -> (-11.8763, 88.8732) centre (-11.5556, 87.926) ccw construction
  arc A149 (-13.4826, 88.8742) -> (-11.8763, 88.8732) centre (-12.6781, 91.2412) ccw construction
  arc A150 (-13.4826, 88.8742) -> (-14.1291, 88.8732) centre (-13.8045, 87.9274) ccw construction
  arc A151 (-15.0478, 89.793) -> (-14.1291, 88.8732) centre (-14.5884, 89.3331) ccw construction
  arc A152 (-15.0478, 89.793) -> (-15.046, 90.4394) centre (-15.9932, 90.1187) ccw construction
  arc A153 (-15.0451, 92.0457) -> (-15.046, 90.4394) centre (-12.6781, 91.2412) ccw construction
  arc A154 (-15.0451, 92.0457) -> (-15.0461, 92.6921) centre (-15.9919, 92.3675) ccw construction
  arc A155 (-14.1263, 93.6108) -> (-15.0461, 92.6921) centre (-14.5862, 93.1515) ccw construction
  line L191 (-57.9836, 100.7939) -> (-57.9765, 106.7939) projected
  line L192 (-70.8407, 100.8091) -> (-57.9836, 100.7939) projected
  line L193 (-58.1024, 100.7298) -> (-70.9595, 100.7298) projected
  line L194 (-70.9595, 100.7298) -> (-2.6725, 100.7298) construction
  line L195 (-70.9595, 100.7298) -> (-2.6725, 100.7298) construction
  line L196 (-22.6725, 60.7298) -> (-2.6725, 60.7298)
  line L197 (-2.6725, 60.7298) -> (-2.6725, 100.7298)
  line L198 (-2.6725, 100.7298) -> (-22.6725, 100.7298)
  line L199 (-22.6725, 100.7298) -> (-22.6725, 60.7298)
  line L200 (-22.6725, -60.7298) -> (-2.6725, -60.7298)
  line L201 (-2.6725, -60.7298) -> (-2.6725, -100.7298)
  line L202 (-2.6725, -100.7298) -> (-22.6725, -100.7298)
  line L203 (-22.6725, -100.7298) -> (-22.6725, -60.7298)
  line L204 (17.3275, -173.8636) -> (17.3275, 176.1364) construction
  line L205 (-22.6725, -173.8636) -> (-22.6725, 176.1364) construction
  line L206 (17.3275, -173.8636) -> (-22.6725, 176.1364) construction
  circle A156 centre (-2.6725, 1.1364) radius 1.55
  circle A157 centre (-2.6725, 51.1364) radius 1.55
  circle A158 centre (-2.6725, 101.1364) radius 1.55
  circle A159 centre (-2.6725, 151.1364) radius 1.55
  circle A160 centre (-2.6725, 201.1364) radius 1.55
  circle A161 centre (-2.6725, -48.8636) radius 1.55
  circle A162 centre (-2.6725, 1.1364) radius 1.55
  circle A163 centre (-2.6725, 51.1364) radius 1.55
  circle A164 centre (-2.6725, 101.1364) radius 1.55
  circle A165 centre (-2.6725, 151.1364) radius 1.55
  circle A166 centre (-2.6725, -98.8636) radius 1.55
  circle A167 centre (-2.6725, -48.8636) radius 1.55
  circle A168 centre (-2.6725, 1.1364) radius 1.55
  circle A169 centre (-2.6725, 51.1364) radius 1.55
  circle A170 centre (-2.6725, 101.1364) radius 1.55
  circle A171 centre (-2.6725, -148.8636) radius 1.55
  circle A172 centre (-2.6725, -98.8636) radius 1.55
  circle A173 centre (-2.6725, -48.8636) radius 1.55
  circle A174 centre (-2.6725, 1.1364) radius 1.55
  circle A175 centre (-2.6725, 51.1364) radius 1.55
  circle A176 centre (-2.6725, -198.8636) radius 1.55
  circle A177 centre (-2.6725, -148.8636) radius 1.55
  circle A178 centre (-2.6725, -98.8636) radius 1.55
  circle A179 centre (-2.6725, -48.8636) radius 1.55
  circle A180 centre (-2.6725, 1.1364) radius 1.55
  line L207 (-113.1024, -174.1661) -> (-113.1024, -179.1661) construction
  line L208 (-93.1024, -179.1661) -> (-113.1024, -179.1661) construction
  line L209 (-93.1024, -174.1661) -> (-113.1024, -174.1661) construction
  circle A181 centre (104.2556, -141.9298) radius 1.5 projected
  line L210 (71.1919, -138.9298) -> (71.1919, -144.9298) projected
  line L211 (71.1919, -144.9298) -> (57.9061, -144.9298) projected
  line L212 (57.9061, -144.9298) -> (57.9061, -138.9298) projected
  line L213 (57.9061, -138.9298) -> (71.1919, -138.9298) projected
  line L214 (97.7633, -55.9298) -> (97.7633, -61.9298) projected
  line L215 (97.7633, -61.9298) -> (84.4776, -61.9298) projected
  line L216 (84.4776, -61.9298) -> (84.4776, -55.9298) projected
  line L217 (84.4776, -55.9298) -> (97.7633, -55.9298) projected
  circle A182 centre (77.5336, -58.9298) radius 1.5 projected
  line L218 (101.4061, -113.2631) -> (101.4061, -87.5965) projected
  line L219 (101.4061, -87.5965) -> (107.4061, -87.5965) projected
  line L220 (107.4061, -87.5965) -> (107.4061, -113.2631) projected
  line L221 (107.4061, -113.2631) -> (101.4061, -113.2631) projected
  line L222 (-83.8167, -100.7298) -> (-83.8167, -106.7298) projected
  line L223 (-83.8167, -106.7298) -> (-96.6738, -106.7298) projected
  line L224 (-96.6738, -106.7298) -> (-96.6738, -100.7298) projected
  line L225 (-96.6738, -100.7298) -> (-83.8167, -100.7298) projected
  line L226 (-109.531, -100.7298) -> (-109.531, -106.7298) projected
  line L227 (-109.531, -106.7298) -> (-122.3881, -106.7298) projected
  line L228 (-122.3881, -106.7298) -> (-122.3881, -100.7298) projected
  line L229 (-122.3881, -100.7298) -> (-109.531, -100.7298) projected
  circle A183 centre (-77.3881, -103.7298) radius 1.5 projected
  circle A184 centre (-129.1261, -141.9298) radius 1.5 projected
  line L230 (84.4776, 138.9298) -> (84.4776, 144.9298) projected
  line L231 (84.4776, 144.9298) -> (97.7633, 144.9298) projected
  line L232 (97.7633, 144.9298) -> (97.7633, 138.9298) projected
  line L233 (97.7633, 138.9298) -> (84.4776, 138.9298) projected
  line L234 (71.1919, 55.9298) -> (57.9061, 55.9298) projected
  line L235 (57.9061, 55.9298) -> (57.9061, 61.9298) projected
  line L236 (57.9061, 61.9298) -> (71.1919, 61.9298) projected
  line L237 (71.1919, 61.9298) -> (71.1919, 55.9298) projected
  circle A185 centre (77.5336, 141.9298) radius 1.5 projected
  line L238 (-135.2452, 100.7298) -> (-148.1024, 100.7298) projected
  line L239 (-148.1024, 100.7298) -> (-148.1024, 106.7298) projected
  line L240 (-148.1024, 106.7298) -> (-135.2452, 106.7298) projected
  line L241 (-135.2452, 106.7298) -> (-135.2452, 100.7298) projected
  line L242 (-70.9595, 106.7298) -> (-58.1024, 106.7298) projected
  line L243 (-58.1024, 106.7298) -> (-58.1024, 100.7298) projected
  line L244 (-58.1024, 100.7298) -> (-70.9595, 100.7298) projected
  line L245 (-70.9595, 100.7298) -> (-70.9595, 106.7298) projected
  circle A186 centre (-77.3881, 141.9298) radius 1.5 projected
  line L246 (-122.3881, 106.7298) -> (-109.531, 106.7298) projected
  line L247 (-109.531, 106.7298) -> (-109.531, 100.7298) projected
  line L248 (-109.531, 100.7298) -> (-122.3881, 100.7298) projected
  line L249 (-122.3881, 100.7298) -> (-122.3881, 106.7298) projected
  line L250 (-96.6738, 100.7298) -> (-96.6738, 106.7298) projected
  line L251 (-96.6738, 106.7298) -> (-83.8167, 106.7298) projected
  line L252 (-83.8167, 106.7298) -> (-83.8167, 100.7298) projected
  line L253 (-83.8167, 100.7298) -> (-96.6738, 100.7298) projected
  circle A187 centre (-103.2571, 141.9298) radius 1.5 projected
  line L254 (-135.2452, 146.1831) -> (-135.2452, 140.1831) projected
  line L255 (-135.2452, 140.1831) -> (-148.1024, 140.1831) projected
  line L256 (-148.1024, 140.1831) -> (-148.1024, 146.1831) projected
  line L257 (-148.1024, 146.1831) -> (-135.2452, 146.1831) projected
  circle A188 centre (77.5336, 58.9298) radius 1.5 projected
  circle A189 centre (104.2556, 141.9298) radius 1.5 projected
  line L258 (107.4061, 113.2631) -> (107.4061, 87.5965) projected
  line L259 (107.4061, 87.5965) -> (101.4061, 87.5965) projected
  line L260 (101.4061, 87.5965) -> (101.4061, 113.2631) projected
  line L261 (101.4061, 113.2631) -> (107.4061, 113.2631) projected
  line L262 (111.049, 138.9298) -> (111.049, 144.9298) projected
  line L263 (111.049, 144.9298) -> (124.3347, 144.9298) projected
  line L264 (124.3347, 144.9298) -> (124.3347, 138.9298) projected
  line L265 (124.3347, 138.9298) -> (111.049, 138.9298) projected
  circle A190 centre (-129.1261, -103.7298) radius 1.5 projected
  circle A191 centre (-77.3881, -141.9298) radius 1.5 projected
  line L266 (-96.6738, -138.9298) -> (-83.8167, -138.9298) projected
  line L267 (-83.8167, -138.9298) -> (-83.8167, -144.9298) projected
  line L268 (-83.8167, -144.9298) -> (-96.6738, -144.9298) projected
  line L269 (-96.6738, -144.9298) -> (-96.6738, -138.9298) projected
  line L270 (-135.2452, -100.7298) -> (-135.2452, -106.7298) projected
  line L271 (-135.2452, -106.7298) -> (-148.1024, -106.7298) projected
  line L272 (-148.1024, -106.7298) -> (-148.1024, -100.7298) projected
  line L273 (-148.1024, -100.7298) -> (-135.2452, -100.7298) projected
  line L274 (150.9061, -55.9298) -> (150.9061, -61.9298) projected
  line L275 (150.9061, -61.9298) -> (137.6204, -61.9298) projected
  line L276 (137.6204, -61.9298) -> (137.6204, -55.9298) projected
  line L277 (137.6204, -55.9298) -> (150.9061, -55.9298) projected
  circle A192 centre (104.2556, -58.9298) radius 1.5 projected
  circle A193 centre (130.9776, -141.9298) radius 1.5 projected
  circle A194 centre (77.5336, -141.9298) radius 1.5 projected
  line L278 (124.3347, -55.9298) -> (124.3347, -61.9298) projected
  line L279 (124.3347, -61.9298) -> (111.049, -61.9298) projected
  line L280 (111.049, -61.9298) -> (111.049, -55.9298) projected
  line L281 (111.049, -55.9298) -> (124.3347, -55.9298) projected
  line L282 (124.3347, -138.9298) -> (124.3347, -144.9298) projected
  line L283 (124.3347, -144.9298) -> (111.049, -144.9298) projected
  line L284 (111.049, -144.9298) -> (111.049, -138.9298) projected
  line L285 (111.049, -138.9298) -> (124.3347, -138.9298) projected
  line L286 (97.7633, -144.9298) -> (84.4776, -144.9298) projected
  line L287 (84.4776, -144.9298) -> (84.4776, -138.9298) projected
  line L288 (84.4776, -138.9298) -> (97.7633, -138.9298) projected
  line L289 (97.7633, -138.9298) -> (97.7633, -144.9298) projected
  line L290 (-135.2452, -146.1831) -> (-148.1024, -146.1831) projected
  line L291 (-148.1024, -146.1831) -> (-148.1024, -140.1831) projected
  line L292 (-148.1024, -140.1831) -> (-135.2452, -140.1831) projected
  line L293 (-135.2452, -140.1831) -> (-135.2452, -146.1831) projected
  line L294 (-70.9595, -144.9298) -> (-70.9595, -138.9298) projected
  line L295 (-70.9595, -138.9298) -> (-58.1024, -138.9298) projected
  line L296 (-58.1024, -138.9298) -> (-58.1024, -144.9298) projected
  line L297 (-58.1024, -144.9298) -> (-70.9595, -144.9298) projected
  circle A195 centre (-103.2571, -103.7298) radius 1.5 projected
  line L298 (137.6204, 144.9298) -> (150.9061, 144.9298) projected
  line L299 (150.9061, 144.9298) -> (150.9061, 138.9298) projected
  line L300 (150.9061, 138.9298) -> (137.6204, 138.9298) projected
  line L301 (137.6204, 138.9298) -> (137.6204, 144.9298) projected
  line L302 (71.1919, 138.9298) -> (57.9061, 138.9298) projected
  line L303 (57.9061, 138.9298) -> (57.9061, 144.9298) projected
  line L304 (57.9061, 144.9298) -> (71.1919, 144.9298) projected
  line L305 (71.1919, 144.9298) -> (71.1919, 138.9298) projected
  line L306 (84.4776, 55.9298) -> (84.4776, 61.9298) projected
  line L307 (84.4776, 61.9298) -> (97.7633, 61.9298) projected
  line L308 (97.7633, 61.9298) -> (97.7633, 55.9298) projected
  line L309 (97.7633, 55.9298) -> (84.4776, 55.9298) projected
  circle A196 centre (104.2556, 58.9298) radius 1.5 projected
  line L310 (-58.1024, 144.9298) -> (-58.1024, 138.9298) projected
  line L311 (-58.1024, 138.9298) -> (-70.9595, 138.9298) projected
  line L312 (-70.9595, 138.9298) -> (-70.9595, 144.9298) projected
  line L313 (-70.9595, 144.9298) -> (-58.1024, 144.9298) projected
  circle A197 centre (-129.1261, 141.9298) radius 1.5 projected
  circle A198 centre (-103.2571, 103.7298) radius 1.5 projected
  line L314 (-109.531, 144.9298) -> (-109.531, 138.9298) projected
  line L315 (-109.531, 138.9298) -> (-122.3881, 138.9298) projected
  line L316 (-122.3881, 138.9298) -> (-122.3881, 144.9298) projected
  line L317 (-122.3881, 144.9298) -> (-109.531, 144.9298) projected
  circle A199 centre (-77.3881, 103.7298) radius 1.5 projected
  circle A200 centre (-129.1261, 103.7298) radius 1.5 projected
  line L318 (-83.8167, 144.9298) -> (-83.8167, 138.9298) projected
  line L319 (-83.8167, 138.9298) -> (-96.6738, 138.9298) projected
  line L320 (-96.6738, 138.9298) -> (-96.6738, 144.9298) projected
  line L321 (-96.6738, 144.9298) -> (-83.8167, 144.9298) projected
  circle A201 centre (130.9776, 141.9298) radius 1.5 projected
  line L322 (124.3347, 55.9298) -> (111.049, 55.9298) projected
  line L323 (111.049, 55.9298) -> (111.049, 61.9298) projected
  line L324 (111.049, 61.9298) -> (124.3347, 61.9298) projected
  line L325 (124.3347, 61.9298) -> (124.3347, 55.9298) projected
  circle A202 centre (130.9776, 58.9298) radius 1.5 projected
  line L326 (150.9061, 55.9298) -> (137.6204, 55.9298) projected
  line L327 (137.6204, 55.9298) -> (137.6204, 61.9298) projected
  line L328 (137.6204, 61.9298) -> (150.9061, 61.9298) projected
  line L329 (150.9061, 61.9298) -> (150.9061, 55.9298) projected
  circle A203 centre (-103.2571, -141.9298) radius 1.5 projected
  line L330 (-58.1024, -106.7298) -> (-70.9595, -106.7298) projected
  line L331 (-70.9595, -106.7298) -> (-70.9595, -100.7298) projected
  line L332 (-70.9595, -100.7298) -> (-58.1024, -100.7298) projected
  line L333 (-58.1024, -100.7298) -> (-58.1024, -106.7298) projected
  line L334 (-109.531, -144.9298) -> (-122.3881, -144.9298) projected
  line L335 (-122.3881, -144.9298) -> (-122.3881, -138.9298) projected
  line L336 (-122.3881, -138.9298) -> (-109.531, -138.9298) projected
  line L337 (-109.531, -138.9298) -> (-109.531, -144.9298) projected
  line L338 (71.1919, -61.9298) -> (57.9061, -61.9298) projected
  line L339 (57.9061, -61.9298) -> (57.9061, -55.9298) projected
  line L340 (57.9061, -55.9298) -> (71.1919, -55.9298) projected
  line L341 (71.1919, -55.9298) -> (71.1919, -61.9298) projected
  line L342 (137.6204, -138.9298) -> (150.9061, -138.9298) projected
  line L343 (150.9061, -138.9298) -> (150.9061, -144.9298) projected
  line L344 (150.9061, -144.9298) -> (137.6204, -144.9298) projected
  line L345 (137.6204, -144.9298) -> (137.6204, -138.9298) projected
  circle A204 centre (130.9776, -58.9298) radius 1.5 projected
  circle A205 centre (0, 0) radius 240 projected
  line L346 (-93.1024, -174.1661) -> (-93.1024, -179.1661) construction
  line L347 (-93.1024, -179.1661) -> (-113.1024, -174.1661) construction
  line L348 (-94.1024, -181.6661) -> (-112.1024, -181.6661)
  line L349 (-114.1024, -179.6661) -> (-114.1024, -173.6661)
  line L350 (-112.1024, -171.6661) -> (-94.1024, -171.6661)
  line L351 (-92.1024, -173.6661) -> (-92.1024, -179.6661)
  line L352 (-92.1024, -181.6661) -> (-114.1024, -171.6661) construction
  line L353 (-114.1024, -181.6661) -> (-92.1024, -171.6661) construction
  arc A206 (-112.1024, -171.6661) -> (-114.1024, -173.6661) centre (-112.1024, -173.6661) ccw
  arc A207 (-114.1024, -179.6661) -> (-112.1024, -181.6661) centre (-112.1024, -179.6661) ccw
  arc A208 (-94.1024, -181.6661) -> (-92.1024, -179.6661) centre (-94.1024, -179.6661) ccw
  arc A209 (-92.1024, -173.6661) -> (-94.1024, -171.6661) centre (-94.1024, -173.6661) ccw
  point P0 (-7, -28.5)
  point P1 (-7, -78.5)
  point P2 (-7, -128.5)
  point P3 (17, -28.5)
  point P4 (17, -78.5)
  point P5 (17, -128.5)
  point P6 (28.5, -12)
  point P7 (25, -12)
  point P8 (28.5, -7)
  point P9 (78.5, -7)
  point P10 (75, -12)
  point P11 (128.5, -7)
  point P12 (125, -12)
  point P13 (28.5, 17)
  point P14 (25, 12)
  point P15 (78.5, 17)
  point P16 (75, 12)
  point P17 (128.5, 17)
  point P18 (125, 12)
  point P19 (101.5834, -33.4298)
  point P20 (101.5834, 33.4298)
  point P21 (-2.6725, 99.5864)
  point P22 (-4.1682, 100.7298)
  point P23 (-2.6725, -97.3136)
  point P24 (-2.6725, -100.4136)
  point P25 (-103.1024, -176.6661)
  dimension "d160" = 50
  dimension "d163" = 24
  dimension "d166" = 7
  dimension "d167" = 10
  dimension "d168" = 25
  dimension "d169" = 7
  dimension "d172" = 50
  dimension "d175" = 24
  dimension "d178" = 18
  dimension "d179" = 15